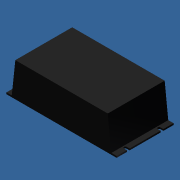
# Autodesk Inventor part: supply-13.8
Saved by Autodesk Inventor 2012 (Build 160160000, 160)
## iProperties
Created: 2012-03-25
Part Number: supply-13.8
Material: Default
Document SubType Name: Modeling
Designer: Edward
Density: 1 g/cm^3
Author: Edward
Autodesk Inventor part; units mm, degrees
ref_plane "YZ Plane" through (0, 0, 0) normal (1, 0, 0) x (0, 1, 0)
ref_plane "XZ Plane" through (0, 0, 0) normal (0, 1, 0) x (-1, 0, 0)
ref_plane "XY Plane" through (0, 0, 0) normal (0, 0, 1) x (1, 0, 0)
sketch "Sketch1" plane through (0, 0, 0) normal (0, 0, 1) x (1, 0, 0)
  line L0 (-98.425, 0) -> (98.425, 0)
  line L1 (98.425, 0) -> (98.425, 2.794)
  line L2 (98.425, 2.794) -> (-98.425, 2.794)
  line L3 (-98.425, 2.794) -> (-98.425, 0)
  line L4 (-88.9, 2.794) -> (-82.55, 60.6044)
  line L5 (-82.55, 60.6044) -> (82.55, 60.6044)
  line L6 (82.55, 60.6044) -> (88.9, 2.794)
  point P0 (0, 0)
  point P1 (0, 0)
  point P2 (0, 2.794)
  point P3 (0, 60.6044)
  dimension "d0" = 196.85
  dimension "d1" = 177.8
  dimension "d2" = 165.1
  dimension "d3" = 2.794
  dimension "d4" = 60.6044
  constraints: 14 end point, 3 midpoint, 2 parallel, 2 perpendicular, 2 point on line, 1 coincident, 1 equal length, 1 horizontal, 1 vertical alignment
  measures "d0" distance of L0.start L0.end
  measures "d1" distance of L4.start L6.end
  measures "d2" distance of L4.end L5.end
  measures "d3" distance between parallel lines of L2 L0
  measures "d4" distance between parallel lines of L0 L5
extrude "Extrusion1" add sketch "Sketch1" along normal blind 101.6
sketch "Sketch2" plane through (-98.425, 0, 0) normal (0, -1, 0) x (1, 0, 0)
  line L0 (196.85, 101.6) -> (0, 101.6) projected
  line L1 (0, 0) -> (0, 101.6) projected
  line L2 (196.85, 0) -> (196.85, 101.6) projected
  line L3 (0, 83.4517) -> (5.207, 83.4517)
  line L4 (5.207, 83.4517) -> (5.207, 78.4733)
  line L5 (5.207, 78.4733) -> (0, 78.4733)
  line L6 (0, 78.4733) -> (0, 83.4517)
  circle A0 centre (5.207, 80.9625) radius 2.4892
  line L7 (0, 50.8) -> (196.85, 50.8)
  line L8 (98.425, 101.6) -> (98.425, 0)
  line L9 (0, 18.1483) -> (5.207, 18.1483)
  line L10 (5.207, 18.1483) -> (5.207, 23.1267)
  line L11 (5.207, 23.1267) -> (0, 23.1267)
  line L12 (0, 23.1267) -> (0, 18.1483)
  circle A1 centre (5.207, 20.6375) radius 2.4892
  line L13 (196.85, 83.4517) -> (191.643, 83.4517)
  line L14 (191.643, 83.4517) -> (191.643, 78.4733)
  line L15 (191.643, 78.4733) -> (196.85, 78.4733)
  line L16 (196.85, 78.4733) -> (196.85, 83.4517)
  circle A2 centre (191.643, 80.9625) radius 2.4892
  line L17 (196.85, 18.1483) -> (191.643, 18.1483)
  line L18 (191.643, 18.1483) -> (191.643, 23.1267)
  line L19 (191.643, 23.1267) -> (196.85, 23.1267)
  line L20 (196.85, 23.1267) -> (196.85, 18.1483)
  circle A3 centre (191.643, 20.6375) radius 2.4892
  dimension "d7" = 4.9784
  dimension "d8" = 5.207
  dimension "d9" = 30.1625
  constraints: 36 end point, 15 symmetric about line, 4 centre point, 4 midpoint, 2 parallel, 2 perpendicular, 1 horizontal, 1 point on line, 1 tangent, 3 other
  measures "d7" diameter of A0
  measures "d8" distance of L3.start L3.end
  measures "d9" distance from line of L7 A0.centre
extrude "Extrusion2" cut sketch "Sketch2" against normal up to next contours L2 L17 A3 L19 | L11 A1 L9 L1 | L2 L15 A2 L13 | A2 L14 | L14 A2 | L3 A0 L5 L1 | A0 L4 | L4 A0 | A1 L10 | L10 A1 | A3 L18 | L18 A3
body "Solid1"
